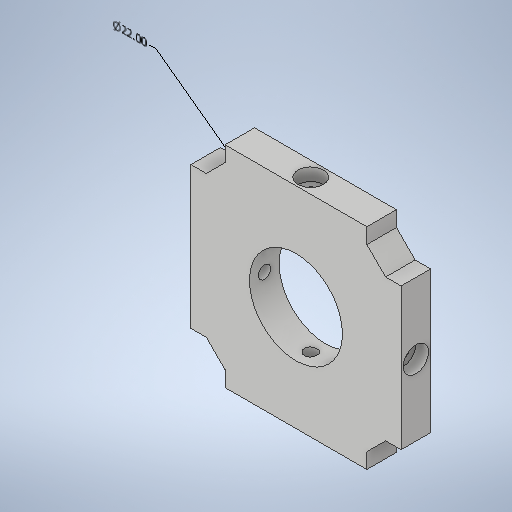
# Autodesk Inventor part: LaserHolder_20mm
Saved by Autodesk Inventor 2025 (Build 290162000, 162)
## iProperties
Created: 2024-08-21
Part Number: LaserHolder_20mm
Material: Generic
Document SubType Name: Sheet Metal
Designer: Administrator
Density: 1 g/cm^3
Sheet Metal Rule: 默认_mm
Appearance: Default
Author: Administrator
Autodesk Inventor part; units mm, degrees
ref_plane "YZ Plane" through (0, 0, 0) normal (1, 0, 0) x (0, 1, 0)
ref_plane "XZ Plane" through (0, 0, 0) normal (0, 1, 0) x (-1, 0, 0)
ref_plane "XY Plane" through (0, 0, 0) normal (0, 0, 1) x (1, 0, 0)
sketch "草图1" plane through (0, 0, 0) normal (0, 0, 1) x (1, 0, 0)
  line L0 (24.9, 16.8) -> (24.9, 0)
  line L1 (24.9, 0) -> (24.9, -16.8)
  line L2 (24.9, 0) -> (41.7, 0) construction
  line L3 (24.9, -16.8) -> (21.24, -16.8)
  line L4 (24.9, 16.8) -> (21.24, 16.8)
  line L5 (-16.8, 24.9) -> (0, 24.9)
  line L6 (0, 24.9) -> (16.8, 24.9)
  line L7 (16.8, 24.9) -> (16.8, 21.24)
  line L8 (-16.8, 24.9) -> (-16.8, 21.24)
  line L9 (-24.9, -16.8) -> (-24.9, 0)
  line L10 (-24.9, 0) -> (-24.9, 16.8)
  line L11 (-24.9, 0) -> (-41.7, 0) construction
  line L12 (-24.9, 16.8) -> (-21.24, 16.8)
  line L13 (-24.9, -16.8) -> (-21.24, -16.8)
  line L14 (16.8, -24.9) -> (0, -24.9)
  line L15 (0, -24.9) -> (-16.8, -24.9)
  line L16 (-16.8, -24.9) -> (-16.8, -21.24)
  line L17 (16.8, -24.9) -> (16.8, -21.24)
  line L18 (-21.24, 16.8) -> (-16.8, 21.24)
  line L19 (16.8, 21.24) -> (21.24, 16.8)
  line L20 (21.24, -16.8) -> (16.8, -21.24)
  line L21 (-16.8, -21.24) -> (-21.24, -16.8)
  point P0 (0, 0)
  constraints: 44 end point, 6 perpendicular, 2 horizontal, 2 vertical
extrude "拉伸1" add sketch "草图1" along normal blind 7
sketch "草图2" plane through (-16.8, 24.9, 0) normal (0, 1, 0) x (1, 0, 0)
  line L0 (0, -7) -> (33.6, -7) projected
  point P0 (16.8, -3.5)
hole "孔1" at (0, 24.9, 3.5) direction (0, -1, 0) diameter 2.97 end through all counterbore diameter 6 counterbore depth 3
sketch "草图3" plane through (-16.8, -24.9, 0) normal (0, -1, 0) x (1, 0, 0)
  point P0 (16.8, 3.5)
hole "孔2" at (0, -24.9, 3.5) direction (0, 1, 0) diameter 2.97 end through all counterbore diameter 6 counterbore depth 3
sketch "草图4" plane through (24.9, -16.8, 0) normal (1, 0, 0) x (0, 0, -1)
  point P0 (0, 16.8)
  point P1 (-3.5, 16.8)
hole "孔3" at (24.9, 0, 3.5) direction (-1, 0, 0) diameter 2.97 end through all counterbore diameter 6 counterbore depth 3
sketch "草图5" plane through (-24.9, -16.8, 0) normal (-1, 0, 0) x (0, 0, 1)
  point P0 (0, 16.8)
  point P1 (3.5, 16.8)
hole "孔4" at (-24.9, 0, 3.5) direction (1, 0, 0) diameter 2.97 end through all counterbore diameter 6 counterbore depth 3
sketch "草图6" plane through (0, 0, 0) normal (0, 0, -1) x (-1, 0, 0)
  point P0 (0, 0)
hole "孔5" at (0, 0, 0) direction (0, 0, 1) diameter 22 end through all
equation "\"d53\" = Thickness"
equation "\"BendRadius\" = Thickness"
equation "\"BendReliefWidth\" = Thickness"
equation "\"BendReliefDepth\" = 0.5 * Thickness"
equation "\"CornerReliefSize\" = 4 * Thickness"
equation "\"MinimumRemnant\" = 2 * Thickness"
equation "\"TransitionRadius\" = BendRadius"
equation "\"JacobiRadiusSize\" = BendRadius"
equation "\"Thickness\" = 0.5"
